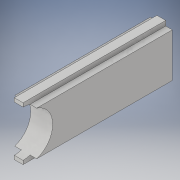
# Autodesk Inventor part: EngineClip
Saved by Autodesk Inventor 2018 (Build 220112000, 112)
## iProperties
Created: 2019-09-13
Part Number: EngineClip
Material: Generic
Document SubType Name: Modeling
Designer: 871357
Density: 1 g/cm^3
Appearance: Default
Author: 871357
Autodesk Inventor part; units mm, degrees
ref_plane "YZ Plane" through (0, 0, 0) normal (1, 0, 0) x (0, 1, 0)
ref_plane "XZ Plane" through (0, 0, 0) normal (0, 1, 0) x (-1, 0, 0)
ref_plane "XY Plane" through (0, 0, 0) normal (0, 0, 1) x (1, 0, 0)
sketch "Sketch1" plane through (0, 0, 0) normal (0, 0, 1) x (1, 0, 0)
  line L0 (12.7, 0) -> (12.7, 25.4)
  line L1 (0, 25.4) -> (0, 0)
  line L2 (3.81, 25.4) -> (8.89, 25.4)
  line L3 (8.89, 25.4) -> (8.89, 28.194)
  line L4 (8.89, 28.194) -> (3.81, 28.194)
  line L5 (3.81, 28.194) -> (3.81, 25.4)
  line L6 (3.81, 0) -> (8.89, 0)
  line L7 (8.89, 0) -> (8.89, -2.794)
  line L8 (8.89, -2.794) -> (3.81, -2.794)
  line L9 (3.81, -2.794) -> (3.81, 0)
  line L10 (12.7, 25.4) -> (8.89, 25.4)
  line L11 (3.81, 25.4) -> (0, 25.4)
  line L12 (0, 0) -> (3.81, 0)
  line L13 (8.89, 0) -> (12.7, 0)
  dimension "d0" = 12.7
  dimension "d1" = 25.4
  dimension "d2" = 5.08
  dimension "d3" = 2.794
  dimension "d4" = 3.81
  dimension "d5" = 5.08
  dimension "d6" = 2.794
  dimension "d7" = 3.81
  constraints: 28 end point, 9 parallel, 4 horizontal, 4 perpendicular
  measures "d0" distance of L1.start L0.end
  measures "d1" distance of L0.end L0.start
  measures "d2" distance of L4.end L3.end
  measures "d3" distance of L3.end L2.end
  measures "d4" distance from line of L1.start L5
  measures "d5" distance of L7.end L8.end
  measures "d6" distance of L6.end L7.end
  measures "d7" distance from line of L1.end L9
extrude "Extrusion1" add sketch "Sketch1" along normal blind 82.55
sketch "Sketch2" plane through (12.7, 0, 0) normal (1, 0, 0) x (0, 0, -1)
  line L0 (-82.55, 25.4) -> (-82.55, 0) projected
  circle A0 centre (-82.55, 12.7) radius 13.335
  point P0 (0, 0)
  dimension "d10" = 26.67
  constraints: 1 centre point, 1 midpoint
  measures "d10" diameter of A0
extrude "Extrusion2" cut sketch "Sketch2" against normal blind 82.55
body "Solid1"
